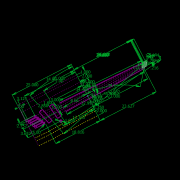
# Autodesk Inventor part: Hybrid
Saved by Autodesk Inventor 2020.4 (Build 244396010, 396A)
## iProperties
Created: 2022-11-06
Part Number: Hybrid
Material: Generic
Document SubType Name: Modeling
Designer: Val
Density: 1 g/cm^3
Appearance: Default
Author: Val
Autodesk Inventor part; units mm, degrees
ref_plane "YZ Plane" through (0, 0, 0) normal (1, 0, 0) x (0, 1, 0)
ref_plane "XZ Plane" through (0, 0, 0) normal (0, 1, 0) x (-1, 0, 0)
ref_plane "XY Plane" through (0, 0, 0) normal (0, 0, 1) x (1, 0, 0)
sketch "SteinbergBoden5" plane through (0, 0, 0) normal (0, 0, 1) x (1, 0, 0)
  line L0 (-265.1838, 66.2948) -> (610.5672, 45.41)
  line L1 (-253.4935, -33.7986) -> (584.2, -11.1347)
  line L2 (610.5672, 45.41) -> (584.2, -11.1347)
  line L3 (-445.5711, 0) -> (780.5345, 0) construction
  line L4 (-265.1838, 66.2948) -> (-253.4935, -33.7986) construction
  line L5 (-330.2, 87.8141) -> (-370.5371, 82.8613)
  line L6 (-370.5371, 82.8613) -> (-353.5119, -55.7974)
  line L7 (-353.5119, -55.7974) -> (-313.1749, -50.8446)
  line L8 (-313.1749, -50.8446) -> (-330.2, 87.8141)
  line L9 (0, -84.2353) -> (0, 115.8314) construction
  line L10 (-442.9271, 87.2481) -> (-482.3599, 77.4164)
  line L11 (-482.3599, 77.4164) -> (-448.5634, -58.1339)
  line L12 (-448.5634, -58.1339) -> (-409.1306, -48.3022)
  line L13 (-409.1306, -48.3022) -> (-442.9271, 87.2481)
  line L14 (-612.775, 70.027) -> (-533.4, 70.027)
  line L15 (-533.4, 70.027) -> (-533.4, 52.247) construction
  line L16 (-533.4, 52.247) -> (-612.775, 52.247)
  line L17 (-612.775, 52.247) -> (-612.775, 70.027)
  circle A0 centre (-533.4, 61.137) radius 8.89
  line L18 (-612.775, 70.027) -> (-630.555, 70.027)
  line L19 (-630.555, 70.027) -> (-630.555, 52.247)
  line L20 (-630.555, 52.247) -> (-612.775, 52.247)
  line L21 (-612.775, 52.247) -> (-612.775, 70.027)
  line L22 (-533.4, 61.137) -> (-477.9163, -57.8481) construction
  line L23 (-635, 228.6) -> (0, 228.6) construction
  line L24 (0, 228.6) -> (0, -209.55) construction
  line L25 (0, -209.55) -> (-635, -209.55) construction
  line L26 (-635, -209.55) -> (-635, 228.6) construction
  line L27 (610.5672, 45.41) -> (643.2113, 45.41)
  line L28 (643.2113, 45.41) -> (643.2113, 38.7509)
  line L29 (643.2113, 38.7509) -> (602.1746, -11.1347)
  line L30 (602.1746, -11.1347) -> (584.2, -11.1347)
  line L31 (-533.4, 61.137) -> (623.244, 37.4869) construction
  line L32 (-521.6688, 35.9793) -> (616.4636, 32.1556) construction
  line L33 (-511.3831, 13.9215) -> (611.3127, 20.8416) construction
  line L34 (-499.7799, -10.9615) -> (605.289, 10.3914) construction
  line L35 (-489.2369, -33.5711) -> (600.1336, -0.0544) construction
  circle A1 centre (-521.6688, 35.9793) radius 8.89
  circle A2 centre (-511.3831, 13.9215) radius 8.89
  circle A3 centre (-499.7799, -10.9615) radius 8.89
  circle A4 centre (-489.2369, -33.5711) radius 8.89
  circle A5 centre (-337.8933, -92.7495) radius 12.7
  line L36 (0, 203.2) -> (-635, 203.2) construction
  line L37 (-635, 203.2) -> (-635, -158.75) construction
  line L38 (-635, -158.75) -> (0, -158.75) construction
  line L39 (0, -158.75) -> (0, 203.2) construction
  line L40 (-635, -127) -> (0, -127) construction
  line L41 (0, -127) -> (0, 152.4) construction
  line L42 (0, 152.4) -> (-635, 152.4) construction
  line L43 (-635, 152.4) -> (-635, -127) construction
  line L44 (-521.6688, 44.8693) -> (-601.0438, 44.8693)
  line L45 (-601.0438, 44.8693) -> (-601.0438, 27.0893)
  line L46 (-601.0438, 27.0893) -> (-521.6688, 27.0893)
  line L47 (-521.6688, 27.0893) -> (-521.6688, 44.8693) construction
  line L48 (-601.0438, 44.8693) -> (-618.8238, 44.8693)
  line L49 (-618.8238, 44.8693) -> (-618.8238, 27.0893)
  line L50 (-618.8238, 27.0893) -> (-601.0438, 27.0893)
  line L51 (-601.0438, 27.0893) -> (-601.0438, 44.8693)
  line L52 (-511.3831, 22.8115) -> (-590.7581, 22.8115)
  line L53 (-590.7581, 22.8115) -> (-590.7581, 5.0315)
  line L54 (-590.7581, 5.0315) -> (-511.3831, 5.0315)
  line L55 (-511.3831, 5.0315) -> (-511.3831, 22.8115) construction
  line L56 (-590.7581, 22.8115) -> (-608.5381, 22.8115)
  line L57 (-608.5381, 22.8115) -> (-608.5381, 5.0315)
  line L58 (-608.5381, 5.0315) -> (-590.7581, 5.0315)
  line L59 (-590.7581, 5.0315) -> (-590.7581, 22.8115)
  line L60 (-499.7799, -2.0715) -> (-579.1549, -2.0715)
  line L61 (-579.1549, -2.0715) -> (-579.1549, -19.8515)
  line L62 (-579.1549, -19.8515) -> (-499.7799, -19.8515)
  line L63 (-499.7799, -19.8515) -> (-499.7799, -2.0715) construction
  line L64 (-579.1549, -2.0715) -> (-596.9349, -2.0715)
  line L65 (-596.9349, -2.0715) -> (-596.9349, -19.8515)
  line L66 (-596.9349, -19.8515) -> (-579.1549, -19.8515)
  line L67 (-579.1549, -19.8515) -> (-579.1549, -2.0715)
  line L68 (-489.2369, -24.6811) -> (-568.6119, -24.6811)
  line L69 (-568.6119, -24.6811) -> (-568.6119, -42.4611)
  line L70 (-568.6119, -42.4611) -> (-489.2369, -42.4611)
  line L71 (-489.2369, -42.4611) -> (-489.2369, -24.6811)
  line L72 (-568.6119, -24.6811) -> (-586.3919, -24.6811)
  line L73 (-586.3919, -24.6811) -> (-586.3919, -42.4611)
  line L74 (-586.3919, -42.4611) -> (-568.6119, -42.4611)
  line L75 (-568.6119, -42.4611) -> (-568.6119, -24.6811)
  point P0 (0, 0)
  point P1 (-462.6435, 82.3322)
  dimension "d155" = 876
  dimension "d156" = 838
  dimension "d157" = 115
  dimension "d158" = 584.2
  dimension "d159" = 7
  dimension "d160" = 139.7
  dimension "d161" = 40.64
  dimension "d162" = 14
  dimension "d163" = 17.78
  dimension "d164" = 17.78
  dimension "d165" = 79.375
  dimension "d166" = 25.4
  dimension "d167" = 635
  dimension "d168" = 330.2
  dimension "d169" = 72.39
  dimension "d170" = 533.4
  dimension "d171" = 25
  dimension "d172" = 25.4
  dimension "d173" = 50.8
  dimension "d174" = 152.4
  dimension "d175" = 127
  dimension "d176" = 31.75
  dimension "d177" = 50.8
  dimension "d178" = 91.366
  dimension "d179" = 91.55
  dimension "d180" = 39.441
  dimension "d181" = 88.238
  dimension "d182" = 88.893
  dimension "d183" = 90.353
  dimension "d184" = 89.808
  dimension "d185" = 88.829
  dimension "d186" = 6.662
  dimension "d187" = 70.027
  dimension "d188" = 643.2113
  dimension "d189" = 45.41
  dimension "d190" = 130.6695
  dimension "d191" = 5.4935
  dimension "d192" = 13.775
  dimension "d193" = 21.8843
  dimension "d194" = 31.6042
  dimension "d195" = 1091.7534
  dimension "d196" = 1166.0124
  dimension "d197" = 623.244
  dimension "d198" = 616.4636
  dimension "d199" = 611.3127
  dimension "d200" = 605.289
  dimension "d201" = 600.1336
  dimension "d202" = 337.8933
  dimension "d203" = 92.7495
  dimension "d204" = 477.9163
  constraints: 152 end point, 31 parallel, 18 perpendicular, 14 horizontal, 10 equal length, 8 collinear, 8 point on circle, 6 centre point, 5 point on line, 5 tangent, 4 coincident, 4 equal radius, 2 midpoint, 2 other
  measures "d155" distance of L4.start L2.start
  measures "d156" distance of L4.end L2.end
  measures "d157" angle of L2 L3
  measures "d158" horizontal distance of L2.end point (0, 0)
  measures "d159" angle of L8 L9
  measures "d160" distance of L7.end L8.end
  measures "d161" distance of L8.end L6.start
  measures "d162" angle of L9 L13
  measures "d163" distance of L16.end L14.start
  measures "d164" distance between parallel lines of L17 L19
  measures "d165" distance of L14.start L15.start
  measures "d166" diameter of A5
  measures "d167" distance of L23.start L24.start
  measures "d168" distance from line of L8.end L9
  measures "d169" horizontal distance of L13.end L6.start
  measures "d170" distance from line of L9 L22.start
  measures "d171" angle of L43 L22
  measures "d172" distance between parallel lines of L36 L23
  measures "d173" distance between parallel lines of L42 L36
  measures "d174" distance between parallel lines of L3 L42
  measures "d175" distance from line of point (0, 0) L40
  measures "d176" distance between parallel lines of L38 L40
  measures "d177" distance between parallel lines of L25 L38
  measures "d178" angle of L9 L0
  measures "d179" angle of L24 L1
  measures "d180" angle of L29 L9
  measures "d181" angle of L35 L9
  measures "d182" angle of L34 L9
  measures "d183" angle of L33 L9
  measures "d184" angle of L32 L9
  measures "d185" angle of L31 L9
  measures "d186" angle of L4 L9
  measures "d187" distance between parallel lines of L3 L14
  measures "d188" distance between parallel lines of L28 L9
  measures "d189" distance between parallel lines of L27 L3
  measures "d190" distance from line of L3.end L29
  measures "d191" distance from line of L3.end L35
  measures "d192" distance from line of L3.end L34
  measures "d193" distance from line of L3.end L33
  measures "d194" distance from line of L3.end L32
  measures "d195" distance from line of L3.end L8
  measures "d196" distance from line of L3.end L13
  measures "d197" distance from line of L31.end L9
  measures "d198" distance from line of L32.end L9
  measures "d199" distance from line of L33.end L9
  measures "d200" distance from line of L34.end L9
  measures "d201" distance from line of L35.end L9
  measures "d202" distance from line of A5.centre L9
  measures "d203" distance from line of A5.centre L3
  measures "d204" distance from line of L22.end L9
sketch "Base" plane through (0, 0, 0) normal (0, 0, 1) x (1, 0, 0)
  line L0 (-572.212, -26.493) -> (-572.212, -44.273) projected
  line L1 (-253.4935, -26.7585) -> (-311.0788, -28.3165)
  line L2 (-268.7156, 45.41) -> (-306.2864, -35.1608)
  line L3 (-254.4055, 79.2682) -> (-234.8574, 45.41)
  line L4 (-254.4055, 79.2682) -> (-127.1182, 193.8782)
  line L5 (-366.1655, 119.38) -> (-394.7405, 119.38)
  line L6 (-366.1655, 119.38) -> (-235.4706, 237.0582)
  line L7 (-235.4706, 237.0582) -> (-79.1619, 237.0582)
  line L8 (-1016.7466, 0) -> (1080.0814, 0) construction
  line L9 (-127.1182, 193.8782) -> (-98.5432, 193.8782)
  line L10 (-98.5432, 193.8782) -> (59.4128, 95.1764)
  line L11 (-79.1619, 237.0582) -> (178.5342, 76.0318) construction
  line L12 (59.4128, 95.1764) -> (41.2993, 45.41)
  line L13 (607.2844, 45.41) -> (584.2, -4.0946)
  line L14 (-127.1182, 193.8782) -> (-79.1619, 237.0582) construction
  line L15 (-394.7405, 119.38) -> (-562.0945, 245.4903)
  line L16 (-535.4156, 88.9) -> (-573.5156, 88.9)
  line L17 (-573.5156, 88.9) -> (-717.1997, -54.7841)
  line L18 (-717.1997, -54.7841) -> (-717.1997, -92.8841)
  line L19 (-460.324, -128.5466) -> (-495.2112, -203.3623)
  line L20 (-495.2112, -203.3623) -> (-401.0074, -217.4411)
  line L21 (-401.0074, -217.4411) -> (-234.0691, -113.1265)
  line L22 (-572.212, 67.6556) -> (-572.212, -44.273)
  line L23 (-572.212, -44.273) -> (-594.6517, -80.1841)
  line L24 (-594.6517, -80.1841) -> (-634.6497, -80.1841)
  line L25 (-634.6497, -80.1841) -> (-634.6497, 27.7659)
  line L26 (-634.6497, 27.7659) -> (-573.5156, 88.9)
  line L27 (-491.4215, 114.3) -> (-535.4156, 88.9)
  line L28 (-717.1997, -92.8841) -> (-507.6497, -92.8841)
  line L29 (-507.6497, -92.8841) -> (-460.324, -128.5466)
  line L30 (-572.212, 67.6556) -> (-535.4156, 88.9) construction
  line L31 (-491.4215, 114.3) -> (-491.4215, 127)
  line L32 (-562.0945, 245.4903) -> (-595.0901, 226.4403)
  line L33 (-491.4215, 127) -> (-595.0901, 226.4403)
  line L34 (-166.5864, -24.4072) -> (-166.5864, -37.1072)
  line L35 (-166.5864, -37.1072) -> (-177.3209, -60.1275)
  line L36 (-177.3209, -60.1275) -> (-110.0071, -102.1898)
  line L37 (-234.0691, -113.1265) -> (-150.4287, -165.3908)
  line L38 (-128.883, -119.1857) -> (-150.4287, -165.3908)
  line L39 (-110.0071, -102.1898) -> (-128.883, -119.1857)
  line L40 (178.5342, 76.0318) -> (178.5342, 45.41)
  line L41 (607.2844, 45.41) -> (658.0844, 45.41)
  line L42 (584.2, -4.0946) -> (635, -4.0946)
  line L43 (658.0844, 45.41) -> (635, -4.0946)
  line L44 (-79.1619, 237.0582) -> (-70.7037, 237.0582)
  line L45 (-70.7037, 237.0582) -> (-70.7037, 224.3582)
  line L46 (-70.7037, 224.3582) -> (166.6681, 76.0318)
  line L47 (166.6681, 76.0318) -> (178.5342, 76.0318)
  line L48 (-288.0278, -109.4047) -> (-277.3953, -86.6032)
  line L49 (-277.3953, -86.6032) -> (-284.6797, -76.2)
  line L50 (-284.6797, -76.2) -> (-339.0744, -76.2)
  line L51 (-339.0744, -76.2) -> (-431.7698, -172.1889)
  line L52 (-431.7698, -172.1889) -> (-433.02, -180.5542)
  line L53 (-433.02, -180.5542) -> (-407.899, -184.3086)
  line L54 (-407.899, -184.3086) -> (-288.0278, -109.4047)
  line L55 (-572.212, 67.6556) -> (-573.5156, 88.9)
  point P0 (0, 0)
  dimension "d51" = 88.9
  dimension "d54" = 33.8582
  dimension "d56" = 102
  dimension "d57" = 119.38
  dimension "d58" = 33.8582
  dimension "d59" = 237.0582
  dimension "d60" = 43.18
  dimension "d61" = 148
  dimension "d62" = 28.575
  dimension "d63" = 186.2582
  dimension "d64" = 120.65
  dimension "d65" = 102
  dimension "d66" = 28.575
  dimension "d67" = 111.76
  dimension "d68" = 143
  dimension "d70" = 209.55
  dimension "d73" = 50.8
  dimension "d74" = 30
  dimension "d75" = 38.1
  dimension "d76" = 88.9
  dimension "d77" = 45
  dimension "d78" = 38.1
  dimension "d80" = 304.8
  dimension "d81" = 209.55
  dimension "d83" = 59.2582
  dimension "d84" = 115
  dimension "d85" = 82.55
  dimension "d86" = 8.5
  dimension "d87" = 32
  dimension "d88" = 95.25
  dimension "d89" = 196.85
  dimension "d94" = 82.55
  dimension "d95" = 12.7
  dimension "d96" = 38.1
  dimension "d97" = 12.7
  dimension "d98" = 139.7
  dimension "d99" = 12.7
  dimension "d100" = 25.4
  dimension "d101" = 79.375
  dimension "d102" = 25.4
  dimension "d104" = 50.8
  dimension "d105" = 8.4582
  dimension "d106" = 12.7
  dimension "d107" = 122
  dimension "d113" = 31.75
  dimension "d114" = 31.75
  dimension "d115" = 50.8
  dimension "d116" = 76.2
  dimension "d117" = 12.7
  dimension "d118" = 8.4582
  dimension "d119" = 14
  dimension "d120" = 25.4
  dimension "d145" = 203.2
  constraints: 108 end point, 23 parallel, 5 horizontal, 4 collinear, 3 vertical, 2 perpendicular
  measures "d51" distance of L2.start L2.end
  measures "d54" distance of L2.start L3.end
  measures "d56" angle of L4 L3
  measures "d57" distance between parallel lines of L8 L5
  measures "d58" vertical distance of L3.end L3.start
  measures "d59" distance between parallel lines of L7 L8
  measures "d60" distance between parallel lines of L7 L9
  measures "d61" angle of L10 L9
  measures "d62" distance of L9.end L4.end
  measures "d63" distance of L9.end L10.end
  measures "d64" distance of L10.end L11.end
  measures "d65" angle of L10 L12
  measures "d66" distance of L5.start L5.end
  measures "d67" horizontal distance of L3.start L5.start
  measures "d68" angle of L15 L5
  measures "d70" distance of L5.end L15.end
  measures "d73" distance of L27.start L16.start
  measures "d74" angle of L8 L27
  measures "d75" distance of L16.end L16.start
  measures "d76" distance between parallel lines of L8 L16
  measures "d77" angle of L8 L17
  measures "d78" distance of L17.end L18.end
  measures "d80" horizontal distance of L16.end L2.start
  measures "d81" distance of L18.end L28.end
  measures "d83" distance of L28.end L19.start
  measures "d84" angle of L8 L2
  measures "d85" distance of L19.start L19.end
  measures "d86" angle of L20 L8
  measures "d87" angle of L8 L21
  measures "d88" distance of L19.end L20.end
  measures "d89" distance of L20.end L21.end
  measures "d94" distance between parallel lines of L18 L25
  measures "d95" distance between parallel lines of L28 L24
  measures "d96" distance of L15.end L32.end
  measures "d97" distance of L27.start L31.end
  measures "d98" horizontal distance of L2.end L34.start
  measures "d99" distance of L34.start L34.end
  measures "d100" distance of L34.end L35.end
  measures "d101" distance of L35.end L36.end
  measures "d102" distance of L36.end L38.start
  measures "d104" distance of L13.start L41.end
  measures "d105" distance of L7.end L44.end
  measures "d106" distance of L44.end L45.end
  measures "d107" angle of L23 L24
  measures "d113" distance between parallel lines of L21 L54
  measures "d114" distance between parallel lines of L20 L53
  measures "d115" distance of L21.end L48.end
  measures "d116" distance between parallel lines of L8 L50
  measures "d117" distance of L48.end L49.end
  measures "d118" distance of L51.end L52.end
  measures "d119" angle of L54 L51
  measures "d120" distance of L52.end L53.end
  measures "d145" distance of L16.end L17.end
extrude "BaseFeature" add sketch "Base" along normal blind 50.8 contours L41 L43 L42 L13
sketch "Holes" plane through (0, 0, 50.8) normal (0, 0, 1) x (1, 0, 0)
  line L0 (77.8278, 78.8058) -> (108.003, 78.8058)
  line L1 (108.003, 78.8058) -> (108.003, 53.863)
  line L2 (108.003, 53.863) -> (80.444, 53.863)
  line L3 (77.8278, 56.4792) -> (77.8278, 78.8058)
  line L4 (-235.4706, 237.0582) -> (-366.1655, 119.38) construction
  line L5 (-281.3415, 115.0334) -> (-234.1518, 157.5232)
  line L6 (-234.1518, 157.5232) -> (-216.629, 138.0621)
  line L7 (-216.629, 138.0621) -> (-263.8187, 95.5723)
  line L8 (-263.8187, 95.5723) -> (-281.3415, 115.0334)
  line L9 (-281.3415, 115.0334) -> (-216.629, 138.0621) construction
  line L10 (-234.1518, 157.5232) -> (-263.8187, 95.5723) construction
  line L11 (77.8278, 53.863) -> (80.444, 53.863)
  line L12 (80.444, 53.863) -> (80.444, 56.4792)
  line L13 (80.444, 56.4792) -> (77.8278, 56.4792)
  line L14 (77.8278, 56.4792) -> (77.8278, 53.863)
  line L15 (41.2993, 45.41) -> (-234.8574, 45.41) construction
  line L16 (41.2993, 45.41) -> (178.5342, 45.41) construction
  line L17 (-98.5432, 193.8782) -> (59.4128, 95.1764) construction
  line L18 (178.5342, 76.0318) -> (166.6681, 76.0318) projected
  line L19 (59.4128, 95.1764) -> (178.5342, 76.0318) construction
  line L20 (-254.4055, 79.2682) -> (-127.1182, 193.8782) construction
  line L21 (-254.4055, 79.2682) -> (-127.1182, 193.8782) construction
  line L22 (-254.4055, 79.2682) -> (-263.8187, 95.5723) construction
  line L23 (-234.8574, 45.41) -> (-254.4055, 79.2682) construction
  line L24 (-246.1225, 111.506) -> (-245.0518, 110.3168)
  line L25 (-245.0518, 110.3168) -> (-233.2544, 120.9393)
  line L26 (-233.2544, 120.9393) -> (-234.3251, 122.1285)
  point P0 (-248.9852, 126.5477)
  dimension "d127" = 30.1752
  dimension "d128" = 24.9428
  dimension "d129" = 2.6162
  dimension "d130" = 8.453
  dimension "d131" = 8.453
  dimension "d132" = 18.415
  dimension "d133" = 63.5
  dimension "d134" = 26.1874
  dimension "d135" = 18.415
  dimension "d136" = 23.8125
  dimension "d137" = 23.8125
  dimension "d139" = 15.875
  dimension "d140" = 1.6002
  constraints: 40 end point, 8 parallel, 6 perpendicular, 2 horizontal, 2 midpoint, 2 point on line, 1 coincident, 1 collinear
  measures "d127" distance of L0.start L0.end
  measures "d128" distance of L0.end L1.end
  measures "d129" distance of L3.start L12.end
  measures "d130" distance from line of L19 L0.end
  measures "d131" distance from line of L16 L1.end
  measures "d132" horizontal distance of L17.end L0.start
  measures "d133" distance of L5.start L5.end
  measures "d134" distance of L5.end L6.end
  measures "d135" distance between parallel lines of L20 L7
  measures "d136" distance of L7.end L24.start
  measures "d137" distance of L6.end L26.end
  measures "d139" distance of L24.end L25.end
  measures "d140" distance of L25.end L26.end
chamfer "Chamfer1" [suppressed]
chamfer "Chamfer3" distance 6.35 angle 45 2 edges at (658.0844, 45.41, 25.4) (635, -4.0946, 25.4)
extrude "HolesFeature" cut sketch "Holes" against normal through all contours L0 L1 L2 L12 L13 L3 | L5 L6 L7 L8 | L7 L26 L25 L24
body "Solid1"
